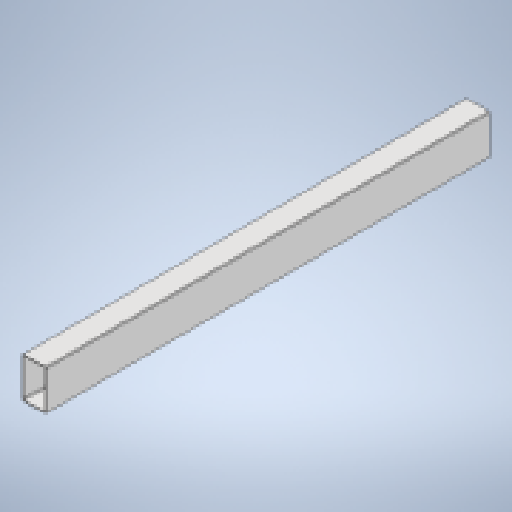
# Autodesk Inventor part: 2x3_Tube
Saved by Autodesk Inventor 2023 (Build 270158000, 158)
## iProperties
Created: 2022-05-03
Part Number: 2x3_Tube
Material: Generic
Document SubType Name: Modeling
Designer: plebbb
Density: 1 g/cm^3
Appearance: Default
Author: plebbb
Autodesk Inventor part; units mm, degrees
ref_plane "YZ Plane" through (0, 0, 0) normal (1, 0, 0) x (0, 1, 0)
ref_plane "XZ Plane" through (0, 0, 0) normal (0, 1, 0) x (-1, 0, 0)
ref_plane "XY Plane" through (0, 0, 0) normal (0, 0, 1) x (1, 0, 0)
sketch "Sketch1" plane through (0, 0, 0) normal (0, 0, 1) x (1, 0, 0)
  line L0 (0, 0) -> (76.2, 0)
  line L1 (76.2, 0) -> (76.2, 127)
  line L2 (76.2, 127) -> (0, 127)
  line L3 (0, 127) -> (0, 0)
  dimension "d0" = 76.2
  dimension "d1" = 127
  constraints: 8 end point, 2 parallel, 1 horizontal, 1 perpendicular
  measures "d0" distance of L1.end L2.end
  measures "d1" distance of L0.end L1.end
extrude "Extrusion1" add sketch "Sketch1" along normal blind 1397
shell "Shell1" thickness 3.175 removed faces 2 at (50.8, 42.3333, 1397) at (50.8, 42.3333, 0)
fillet "Fillet1" radius 3.175 8 edges at (0, 127, 698.5) (3.175, 123.825, 698.5) (76.2, 127, 698.5) (73.025, 123.825, 698.5) (3.175, 3.175, 698.5) (0, 0, 698.5) (76.2, 0, 698.5) (73.025, 3.175, 698.5)
sketch "Sketch2" plane through (6.35, 3.175, 0) normal (0, 1, 0) x (1, 0, 0)
  line L0 (-6.35, 0) -> (69.85, 0)
  line L1 (69.85, 0) -> (69.85, -76.2)
  line L2 (69.85, -76.2) -> (-6.35, -76.2)
  line L3 (-6.35, -76.2) -> (-6.35, 0)
  line L4 (51.75, -11.6) -> (11.75, -11.6) construction
  line L5 (11.75, -11.6) -> (11.75, -64.6) construction
  line L6 (11.75, -64.6) -> (51.75, -64.6)
  line L7 (51.75, -64.6) -> (51.75, -11.6) construction
  circle A0 centre (11.75, -64.6) radius 4
  circle A1 centre (11.75, -11.6) radius 4
  circle A2 centre (51.75, -64.6) radius 4
  circle A3 centre (51.75, -11.6) radius 4
  circle A4 centre (31.75, -38.1) radius 4
  circle A5 centre (31.75, -1358.9) radius 4
  line L8 (51.75, -1332.4) -> (11.75, -1332.4) construction
  line L9 (11.75, -1332.4) -> (11.75, -1385.4) construction
  line L10 (-6.35, -1320.8) -> (69.85, -1320.8)
  line L11 (-6.35, -1397) -> (-6.35, -1320.8)
  circle A6 centre (11.75, -1332.4) radius 4
  line L12 (51.75, -1385.4) -> (51.75, -1332.4) construction
  line L13 (69.85, -1320.8) -> (69.85, -1397)
  circle A7 centre (51.75, -1332.4) radius 4
  line L14 (11.75, -1385.4) -> (51.75, -1385.4)
  circle A8 centre (11.75, -1385.4) radius 4
  line L15 (69.85, -1397) -> (-6.35, -1397)
  circle A9 centre (51.75, -1385.4) radius 4
  point P0 (31.75, -64.6)
  point P1 (31.75, -76.2)
  point P2 (51.75, -38.1)
  point P3 (69.85, -38.1)
  point P4 (51.75, -1358.9)
  point P5 (69.85, -1358.9)
  point P6 (31.75, -1385.4)
  point P7 (31.75, -1397)
  dimension "d6" = 76.2
  dimension "d7" = 76.2
  dimension "d8" = 53
  dimension "d9" = 40
  dimension "d10" = 8
  dimension "d13" = 1320.8
  constraints: 32 end point, 10 centre point, 10 coincident, 4 equal radius, 4 midpoint, 4 parallel, 2 horizontal, 2 horizontal alignment, 2 perpendicular, 2 vertical alignment, 1 collinear, 1 vertical, 30 other
  measures "d6" distance of L0.end L1.end
  measures "d7" distance of L1.end L2.end
  measures "d8" distance of L6.end L4.start
  measures "d9" distance of L5.end L6.end
  measures "d10" diameter of A2
  measures "d13" distance of point (51.75, -38.1) point (51.75, -1358.9)
extrude "Extrusion2" cut sketch "Sketch2" against normal up to surface (3.175 mm away) contours A0 | A1 | A2 | A3 | A4 | A5 | A6 | A7 | A8 | A9
body "Solid1"
